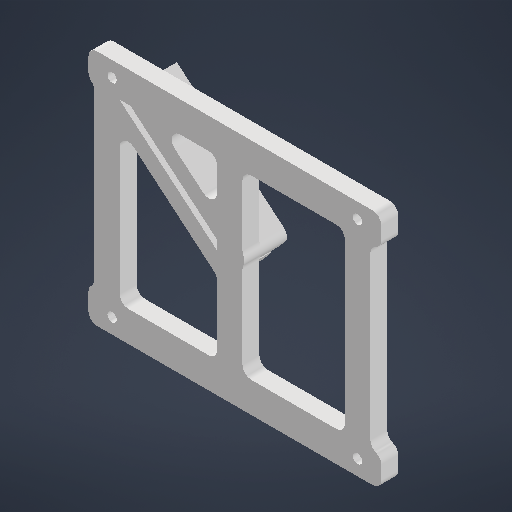
# Autodesk Inventor part: rpi-mount
Saved by Autodesk Inventor 2025 (Build 290162000, 162)
## iProperties
Created: 2024-09-27
Part Number: rpi-mount
Material: Generic
Document SubType Name: Modeling
Designer: Windows 7 was better
Density: 1 g/cm^3
Appearance: Default
Author: Windows 7 was better
Autodesk Inventor part; units mm, degrees
ref_plane "YZ Plane" through (0, 0, 0) normal (1, 0, 0) x (0, 1, 0)
ref_plane "XZ Plane" through (0, 0, 0) normal (0, 1, 0) x (-1, 0, 0)
ref_plane "XY Plane" through (0, 0, 0) normal (0, 0, 1) x (1, 0, 0)
sketch "Sketch1" plane through (0, 0, 0) normal (0, 0, 1) x (1, 0, 0)
  line L0 (35, 0) -> (35, -4)
  line L1 (0, -4) -> (0, 0)
  line L2 (0, 0) -> (0, 1.8) construction
  line L3 (35, 1.8) -> (35, 5.8)
  line L4 (0, 5.8) -> (0, 1.8)
  line L5 (-9.2123, 0.9) -> (-9.2123, 25.4) construction
  line L6 (-9.2123, 25.4) -> (-9.2123, -23.6) construction
  line L7 (-9.2123, -23.6) -> (48.7877, -23.6) construction
  line L8 (-9.2123, 25.4) -> (48.7877, 25.4) construction
  circle A0 centre (48.7877, 25.4) radius 1.1
  circle A1 centre (-9.2123, 25.4) radius 1.1
  circle A2 centre (-9.2123, -23.6) radius 1.1
  circle A3 centre (48.7877, -23.6) radius 1.1
  line L9 (-14.8123, -20) -> (54.3877, -20)
  line L10 (54.3877, -20) -> (54.3877, -27.2)
  line L11 (54.3877, -27.2) -> (-14.8123, -27.2)
  line L12 (-14.8123, -27.2) -> (-14.8123, -20)
  line L13 (-14.8123, -20) -> (54.3877, -27.2) construction
  line L14 (54.3877, -20) -> (-14.8123, -27.2) construction
  line L15 (-14.8123, 29) -> (54.3877, 29)
  line L16 (54.3877, 29) -> (54.3877, 21.8)
  line L17 (54.3877, 21.8) -> (-14.8123, 21.8)
  line L18 (-14.8123, 21.8) -> (-14.8123, 29)
  line L19 (-14.8123, 29) -> (54.3877, 21.8) construction
  line L20 (54.3877, 29) -> (-14.8123, 21.8) construction
  line L21 (21.5942, 21.8) -> (15.5942, 21.8)
  line L22 (15.5942, 21.8) -> (15.5942, -20)
  line L23 (15.5942, -20) -> (21.5942, -20)
  line L24 (21.5942, -20) -> (21.5942, 21.8)
  line L25 (-13.4058, 21.8) -> (-7.4058, 21.8)
  line L26 (-7.4058, 21.8) -> (-7.4058, -20)
  line L27 (-7.4058, -20) -> (-13.4058, -20)
  line L28 (-13.4058, -20) -> (-13.4058, 21.8)
  line L29 (19.7877, 25.4) -> (19.7877, 0) construction
  line L30 (19.7877, 0) -> (-7.0239, 22.4976) construction
  line L31 (-7.0239, 22.4976) -> (-6.4775, 23.1487) construction
  line L32 (-6.4775, 23.1487) -> (-7.5703, 21.8464) construction
  line L33 (-7.5703, 21.8464) -> (19.2413, -0.6511)
  line L34 (19.2413, -0.6511) -> (16.6701, -3.7153)
  line L35 (16.6701, -3.7153) -> (-10.1414, 18.7823)
  line L36 (-10.1414, 18.7823) -> (-7.5703, 21.8464)
  line L37 (-6.4775, 23.1487) -> (20.334, 0.6511)
  line L38 (20.334, 0.6511) -> (22.9052, 3.7153)
  line L39 (22.9052, 3.7153) -> (-3.9064, 26.2129)
  line L40 (-3.9064, 26.2129) -> (-6.4775, 23.1487)
  line L41 (16.6701, -3.7153) -> (15.5942, -2.8125)
  line L42 (-3.9064, 26.2129) -> (-7.4058, 29.1492)
  line L43 (48.7877, 25.4) -> (48.7877, -23.6) construction
  line L44 (51.7877, 25.4) -> (51.7877, -23.6)
  line L45 (51.7877, -23.6) -> (45.7877, -23.6)
  line L46 (45.7877, -23.6) -> (45.7877, 25.4)
  line L47 (45.7877, 25.4) -> (51.7877, 25.4)
  line L48 (51.7877, 25.4) -> (45.7877, -23.6) construction
  line L49 (51.7877, -23.6) -> (45.7877, 25.4) construction
  point P0 (19.7877, -23.6)
  point P1 (15.5942, 21.8)
  point P2 (-13.4058, -20)
  point P3 (21.5942, -20)
  point P4 (15.5942, 9.8499)
  point P5 (-3.5756, 21.5548)
  point P6 (15.5942, 4.6283)
  point P7 (15.5942, 2.4091)
  point P8 (-7.4058, 21.7084)
  point P9 (-3.5756, 18.7941)
  point P10 (19.4244, -5.4852)
  point P11 (-7.4058, 16.4868)
  point P12 (-7.6092, 21.8)
  point P13 (-7.5149, 21.8)
  point P14 (21.5942, 2.153)
  point P15 (1.3527, 21.8)
  point P16 (-4.8702, 21.8)
  point P17 (21.5942, 4.8153)
  point P18 (48.7877, 0.9)
  point P19 (45.7877, 21.8)
  point P20 (45.7877, -20)
  point P21 (51.7877, -20)
  point P22 (51.7877, 21.8)
  dimension "d7" = 24.5
  dimension "d8" = 49
  dimension "d9" = 58
  dimension "d10" = 58
  dimension "d11" = 2.2
  dimension "d12" = 2.2
  dimension "d13" = 2.2
  dimension "d14" = 2.2
  dimension "d15" = 69.2
  dimension "d16" = 7.2
  dimension "d17" = 69.2
  dimension "d18" = 7.2
  dimension "d19" = 6
  dimension "d20" = 6
  dimension "d26" = 35
  dimension "d27" = 50
  dimension "d28" = 0.85
  dimension "d29" = 1.7
  dimension "d30" = 35
  dimension "d31" = 4
  dimension "d32" = 4
  dimension "d36" = 6
  constraints: 100 end point, 18 parallel, 10 perpendicular, 9 midpoint, 9 point on line, 6 horizontal, 4 centre point, 4 coincident, 3 vertical
  measures "d7" distance of L5.start L5.end
  measures "d8" distance of L5.end L6.end
  measures "d9" distance of L6.end L7.end
  measures "d10" distance of L5.end L8.end
  measures "d11" diameter of A0
  measures "d12" diameter of A1
  measures "d13" diameter of A2
  measures "d14" diameter of A3
  measures "d15" distance of L10.end L11.end
  measures "d16" distance of L9.end L10.end
  measures "d17" distance of L16.end L17.end
  measures "d18" distance of L15.end L16.end
  measures "d19" distance of L23.end L22.end
  measures "d20" distance of L26.end L27.end
  measures "d26" distance of L29.end L30.end
  measures "d27" angle of L29 L30
  measures "d28" distance of L30.end L31.end
  measures "d29" distance of L31.end L32.end
  measures "d30" distance of L32.end L33.end
  measures "d31" distance of L33.end L34.end
  measures "d32" distance of L38.end L37.end
  measures "d36" distance of L44.end L45.end
extrude "Extrusion1" add sketch "Sketch1" along normal blind 4 contours L47 L44 L17 L46 A0 | A0 L47 L46 L17 L39 L42 L15 L16 L44 | L44 L9 L46 L17 | L44 L45 A3 L46 L9 | L9 L10 L11 L12 L46 L45 A3 L44 | L24 L39 L22 L17 | L39 L38 L24 | L24 L38 L37 L22 L39 | L9 L22 L35 L34 L33 L37 L38 L24 | L42 L40 L37 L17 L33 L36 L18 L15 | L39 L22 L37 L17 | L17 L37 L40 L39 | L9 L28 L17 L36 L35 L26 | L35 L26 L33 L22 | L22 L33 L34 L35 | L26 L33 L17 | L35 L36 L17 L33 L26 | L17 L36 L33
extrude "Extrusion2" add sketch "Sketch1" against normal blind 6 contours L39 L38 L24 | L24 L38 L37 L22 L39 | L39 L22 L37 L17 | L17 L37 L40 L39 | L35 L26 L33 L22 | L22 L33 L34 L35 | L35 L36 L17 L33 L26 | L17 L36 L33
fillet "Fillet1" radius 2 16 edges at (54.3877, -27.2, 2) (54.3877, -20, 2) (21.5942, -20, 2) (21.5942, 21.8, 2) (54.3877, 21.8, 2) (54.3877, 29, 2) (-14.8123, 29, 2) (-14.8123, 21.8, 2) (-7.4058, 21.8, 2) (15.5942, 21.8, 2) (-13.4058, 21.8, 2) (15.5942, -20, 2) (-7.4058, -20, 2) (-13.4058, -20, 2) (-14.8123, -20, 2) (-14.8123, -27.2, 2)
fillet "Fillet2" radius 2 5 edges at (15.5942, 9.8499, 2) (-7.4058, 16.4868, 2) (22.9052, 3.7153, -1) (15.5942, -2.8125, 2) (1.3527, 21.8, 2)
fillet "Fillet3" radius 2 2 edges at (6.9282, 11.8999, -6) (5.8355, 10.5976, -6)
fillet "Fillet4" radius 2 6 edges at (21.5942, 2.153, 2) (21.5942, 4.784, 2) (51.7877, -20, 2) (51.7877, 21.8, 2) (45.7877, 21.8, 2) (45.7877, -20, 2)
body "Solid1"
